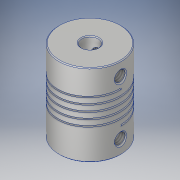
# Autodesk Inventor part: 5mm shaft coupler
Saved by Autodesk Inventor 2018 (Build 220112000, 112)
## iProperties
Created: 2017-11-20
Part Number: 5mm shaft coupler
Material: Aluminum 6061
Document SubType Name: Modeling
Designer: Gabriel Smolnycki
Density: 2.7 g/cm^3
Appearance: Aluminum - Flat
Author: Gabriel Smolnycki
Autodesk Inventor part; units mm, degrees
ref_plane "XZ Plane" through (0, 0, 0) normal (0, 1, 0) x (-1, 0, 0)
ref_plane "XY Plane" through (0, 0, 0) normal (0, 0, 1) x (1, 0, 0)
sketch "Sketch1" plane through (0, 0, 0) normal (0, 1, 0) x (-1, 0, 0)
  circle A0 centre (0, 0) radius 2.5
  circle A1 centre (0, 0) radius 9.4
  dimension "d0" = 5
  dimension "d1" = 18.8
  constraints: 2 centre point, 2 coincident
  measures "d0" diameter of A0
  measures "d1" diameter of A1
extrude "Extrusion1" add sketch "Sketch1" along normal blind 24.8
ref_plane "Work Plane1" through (9.4, 0, 0) normal (1, 0, 0) x (0, 1, 0)
sketch "Sketch2" plane through (9.4, 0, 0) normal (1, 0, 0) x (0, 1, 0)
  line L0 (24.8, 2.5) -> (24.8, -2.5) projected
  point P0 (0, 0)
  point P1 (4.2, 0)
  point P2 (20.6, 0)
  dimension "d4" = 4.2
  dimension "d5" = 4.2
  measures "d4" distance of point (0, 0) point (4.2, 0)
  measures "d5" distance from line of point (20.6, 0) L0
hole "Hole1" at (9.4, 4.2, 0) at (9.4, 20.6, 0) direction (-1, 0, 0) diameter 3.242 depth 9 tip angle 118 countersink diameter 4 countersink angle 90 thread size "M4x0.7" class "6H" standard "ISO Metric profile"
pattern_circular "Circular Pattern1" count 2 over 90 about axis through (0, -10, 0) along (0, 1, 0) of "Hole1"
sketch "Sketch3" plane through (0, 0, 0) normal (0, 0, 1) x (1, 0, 0)
  line L0 (2.5, 0) -> (2.5, 24.8) projected
  line L1 (9.4, 0) -> (9.4, 24.8) projected
  line L2 (2.5, 7.6) -> (9.4, 7.6)
  line L3 (2.5, 8.05) -> (9.4, 8.05)
  line L4 (-9.4, 0) -> (9.4, 0) projected
  line L5 (2.5, 7.6) -> (2.5, 8.05)
  line L6 (9.4, 7.6) -> (9.4, 8.05)
  point P0 (0, 0)
  dimension "d19" = 0.45
  dimension "d20" = 7.6
  constraints: 8 end point, 4 point on line, 2 perpendicular, 1 collinear, 1 horizontal
  measures "d19" distance between parallel lines of L3 L2
  measures "d20" distance between parallel lines of L4 L2
coil "Coil1" sketch "Sketch3" operation cut axis through (0, -10, 0) along (0, 1, 0) pitch 1.92 turns 5 hand right contours L0 L3 L1 L2
chamfer "Chamfer2" distance 0.25 angle 45 4 edges at (2.5, 24.8, 0) (9.4, 24.8, 0) (2.5, 0, 0) (9.4, 0, 0)
equation "\"d5\" = d4"
body "Solid1"
